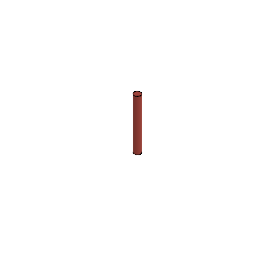
BiggerButton (Autodesk Fusion 360 design; units mm, degrees)
Autodesk Fusion 360 part; units mm, degrees
sketch "Sketch1" plane through (0, 0, 38.77) normal (0, 0, 1) x (-1, 0, 0)
  line L0 (-23.7536, 17.5343) -> (-33.4413, 17.5343)
  arc A0 (-33.4413, 17.5343) -> (-35.9813, 14.9943) centre (-33.4413, 14.9943) ccw
  line L1 (-35.9813, 14.9943) -> (-35.9813, -30.4887)
  arc A1 (-35.9813, -30.4887) -> (-33.4413, -33.0287) centre (-33.4413, -30.4887) ccw
  line L2 (-33.4413, -33.0287) -> (-11.7434, -33.0287)
  arc A2 (-11.7434, -33.0287) -> (-9.2034, -30.4887) centre (-11.7434, -30.4887) ccw
  line L3 (-9.2034, -30.4887) -> (-9.2034, -23.6258)
  arc A3 (-9.2034, -23.6258) -> (-11.7434, -21.0858) centre (-11.7434, -23.6258) ccw
  line L4 (-11.7434, -21.0858) -> (-18.6736, -21.0858)
  arc A4 (-21.2136, -18.5458) -> (-18.6736, -21.0858) centre (-18.6736, -18.5458) ccw
  line L5 (-21.2136, -18.5458) -> (-21.2136, 14.9943)
  arc A5 (-21.2136, 14.9943) -> (-23.7536, 17.5343) centre (-23.7536, 14.9943) ccw
  circle A6 centre (-29.248, -4.071) radius 2.54 construction
  circle A7 centre (-29.245, -16.771) radius 2.54
  circle A8 centre (-24.6385, -1.8886) radius 1.27
  circle A9 centre (-24.6385, -18.4179) radius 1.27
  circle A10 centre (-24.6385, -24.1319) radius 1.27
  circle A11 centre (-29.2419, -29.471) radius 2.54
  circle A12 centre (-17.6852, -28.1982) radius 2.54
  circle A13 centre (-29.248, -4.071) radius 2.54 construction
  circle A14 centre (-29.248, -4.071) radius 3.5577 construction
  circle A15 centre (-29.248, -4.071) radius 2.286
  circle A16 centre (-29.248, -4.071) radius 3.202
  circle A17 centre (-23.7536, 14.9943) radius 1.3
  circle A18 centre (-11.7434, -27.5028) radius 1.3
  dimension "d31" = 5.08
  dimension "d32" = 7.1155
  dimension "d33" = 6.4039
  dimension "d34" = 4.572
  measures "d31" diameter of A6
  measures "d32" diameter of A14
  measures "d33" diameter of A16
  measures "d34" diameter of A15
extrude "Extrude1" add sketch "Sketch1" along normal up to surface (50.076 mm away) from surface at -1.778 contours A15 | A16
extrude "Extrude2" add sketch "Sketch1" along normal blind 2.54 and the other way blind 1.778 contours A15
equation "d33 = 0.280136 in * 0.90"
equation "d34 = 0.20 in * 0.90"
